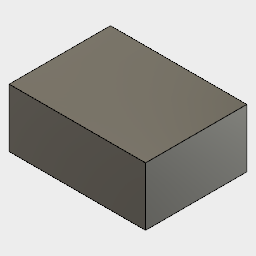
ESC CUBE v1 (Autodesk Fusion 360 design; units mm, degrees)
Autodesk Fusion 360 part; units mm, degrees
sketch "Sketch1" plane through (0, 0, 0) normal (0, 1, 0) x (1, 0, 0)
  line L0 (0, 0) -> (35, 0)
  line L1 (35, 0) -> (35, 26)
  line L2 (35, 26) -> (0, 26)
  line L3 (0, 26) -> (0, 0)
  line L4 (0, 0) -> (0, 3)
  line L5 (0, 0) -> (7.62, 0)
  line L6 (0, 5) -> (0, 0)
  line L7 (0, 0) -> (6, 0)
  line L8 (6, 0) -> (6, 2)
  line L9 (6, 2) -> (0, 2)
  line L10 (0, 2) -> (0, 0)
  line L11 (6, 2) -> (30, 2)
  line L12 (30, 2) -> (30, 23)
  line L13 (30, 23) -> (6, 23)
  line L14 (6, 23) -> (6, 2)
  dimension "d2" = 35
  dimension "d5" = 7.62
  dimension "d7" = 6
  dimension "d8" = 2
  dimension "d9" = 24
  dimension "d10" = 21
  measures "d2" distance of L0.start L0.end
  measures "d5" distance of L0.start L5.end
  measures "d7" distance of L0.start L7.end
  measures "d8" distance of L0.start L9.end
  measures "d9" distance of L8.end L11.end
  measures "d10" distance of L8.end L13.end
extrude "Extrude1" add sketch "Sketch1" along normal blind 15 contours L0 L3 L4 L5 L6 L7 L8 L9 L10 | L11 L12 L13 L14 | L0 L1 L2 L3 L4 L5 L6 L8 L9
